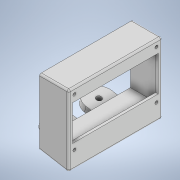
# Autodesk Inventor part: caica display
Saved by Autodesk Inventor 2022 (Build 260153000, 153)
## iProperties
Created: 2022-03-11
Part Number: caica display
Material: Genérico
Document SubType Name: Modeling
Designer: Guilherme
Density: 1 g/cm^3
Appearance: Padrão
Author: Guilherme
Autodesk Inventor part; units mm, degrees
ref_plane "YZ Plane" through (0, 0, 0) normal (1, 0, 0) x (0, 1, 0)
ref_plane "XZ Plane" through (0, 0, 0) normal (0, 1, 0) x (-1, 0, 0)
ref_plane "XY Plane" through (0, 0, 0) normal (0, 0, 1) x (1, 0, 0)
sketch "Esboço1" plane through (0, 0, 0) normal (1, 0, 0) x (0, 1, 0)
  line L0 (-31, 50) -> (31, 50)
  line L1 (31, 50) -> (31, -50)
  line L2 (31, -50) -> (-31, -50)
  line L3 (-31, -50) -> (-31, 50)
  line L4 (-31, 50) -> (31, -50) construction
  line L5 (31, 50) -> (-31, -50) construction
  point P0 (0, 0)
  dimension "d0" = 62
  dimension "d1" = 100
  constraints: 12 end point, 2 midpoint, 2 parallel, 1 horizontal, 1 perpendicular
  measures "d0" distance of L1.end L2.end
  measures "d1" distance of L0.end L1.end
extrude "Extrusão1" add sketch "Esboço1" along normal blind 3
sketch "Esboço4" plane through (0, 0, 0) normal (-1, 0, 0) x (0, 0, 1)
  line L0 (-50, 31) -> (50, 31) projected
  line L1 (-50, -31) -> (50, -31)
  line L2 (50, -31) -> (50, 31)
  line L3 (50, 31) -> (-50, 31)
  line L4 (-50, 31) -> (-50, -31)
  line L5 (-50, -31) -> (50, 31) construction
  line L6 (50, -31) -> (-50, 31) construction
  line L7 (-53, -34) -> (53, -34)
  line L8 (53, -34) -> (53, 34)
  line L9 (53, 34) -> (-53, 34)
  line L10 (-53, 34) -> (-53, -34)
  line L11 (-53, -34) -> (53, 34) construction
  line L12 (53, -34) -> (-53, 34) construction
  point P0 (0, 0)
  dimension "d16" = 106
  dimension "d17" = 68
  constraints: 24 end point, 4 midpoint, 4 parallel, 2 horizontal, 2 perpendicular
  measures "d16" distance of L9.end L8.end
  measures "d17" distance of L8.end L7.end
extrude "Extrusão3" add sketch "Esboço4" along normal blind 30 and the other way blind 3
sketch "Esboço5" plane through (0, 0, 0) normal (-1, 0, 0) x (0, 0, 1)
  line L0 (-49.0345, -29.972) -> (49.0345, -29.972)
  line L1 (49.0345, -29.972) -> (49.0345, 29.972)
  line L2 (49.0345, 29.972) -> (-49.0345, 29.972)
  line L3 (-49.0345, 29.972) -> (-49.0345, -29.972)
  line L4 (-49.0345, -29.972) -> (49.0345, 29.972) construction
  line L5 (49.0345, -29.972) -> (-49.0345, 29.972) construction
  line L6 (-48.55, -20) -> (48.55, -20)
  line L7 (48.55, -20) -> (48.55, 20)
  line L8 (48.55, 20) -> (-48.55, 20)
  line L9 (-48.55, 20) -> (-48.55, -20)
  line L10 (-48.55, -20) -> (48.55, 20) construction
  line L11 (48.55, -20) -> (-48.55, 20) construction
  circle A0 centre (46.4815, 27.305) radius 1.6765
  circle A1 centre (-46.4825, 27.305) radius 1.6765
  circle A2 centre (46.4815, -27.305) radius 1.6765
  circle A3 centre (-46.4825, -27.305) radius 1.6765
  point P0 (0, 0)
  dimension "d22" = 98.069
  dimension "d23" = 59.944
  dimension "d24" = 97.1
  dimension "d25" = 40
  dimension "d26" = 3.353
  dimension "d27" = 2.667
  dimension "d28" = 2.553
  dimension "d31" = 92.964
  dimension "d34" = 54.61
  constraints: 24 end point, 4 centre point, 4 midpoint, 4 parallel, 3 horizontal, 2 perpendicular, 1 vertical, 6 other
  measures "d22" distance of L2.end L1.end
  measures "d23" distance of L1.end L0.end
  measures "d24" distance of L8.end L7.end
  measures "d25" distance of L7.end L6.end
  measures "d26" diameter of A0
  measures "d27" distance from line of L2 A0.centre
  measures "d28" distance from line of L1 A0.centre
  measures "d31" distance of A0.centre A1.centre
  measures "d34" distance of A0.centre A2.centre
extrude "Extrusão4" cut sketch "Esboço5" against normal blind 30 contours L9 L8 L7 L6 | A0 | A1 | A2 | A3
sketch "Esboço20" plane through (-30, 34, 53) normal (0, 0, 1) x (1, 0, 0)
  line L0 (0, -68) -> (0, 0) projected
  line L1 (0, -68) -> (33, -68)
  line L2 (33, -68) -> (33, -75)
  line L3 (0, -75) -> (0, -68)
  line L4 (0, -75) -> (33, -80.8188)
  line L5 (0, -75) -> (34.0016, -75) construction
  line L6 (33, -75) -> (33, -80.8188)
  point P0 (30, -34)
  dimension "d110" = 10
  constraints: 12 end point, 2 horizontal, 2 perpendicular, 1 parallel
  measures "d110" angle of L4 L5
extrude "Extrusão16" add sketch "Esboço20" against normal blind 106
sketch "Esboço23" plane through (-30, 34, 53) normal (0, 0, 1) x (1, 0, 0)
  line L0 (0, 0) -> (0, -75) projected
  line L1 (0, -75) -> (-24.6202, -70.6588)
  line L2 (0, -75) -> (25, -75) construction
  line L3 (-24.6202, -70.6588) -> (-23.4047, -63.7651)
  line L4 (-23.4047, -63.7651) -> (0, -67.892)
  line L5 (0, -67.892) -> (0, -75)
  point P0 (30, -34)
  dimension "d122" = 25
  dimension "d123" = 170
  dimension "d124" = 7
  constraints: 10 end point, 2 perpendicular, 1 equal length, 1 horizontal, 1 point on line, 1 vertical
  measures "d122" distance of L0.end L1.end
  measures "d123" angle of L2 L1
  measures "d124" distance of L1.end L3.end
extrude "Extrusão18" add sketch "Esboço23" against normal blind 106
sketch "Esboço24" plane through (-30, 34, -53) normal (0, 1, 0) x (1, 0, 0)
  line L0 (0, -103) -> (0, -3) projected
  line L1 (0, -15) -> (-28.0822, -15)
  line L2 (-28.0822, -45) -> (0, -45)
  line L3 (0, -45) -> (0, -15)
  line L4 (0, -61) -> (-33.5512, -61)
  line L5 (-33.5512, -91) -> (0, -91)
  line L6 (0, -91) -> (0, -61)
  line L7 (-23.4047, 0) -> (0, 0) projected
  line L8 (0, -106) -> (-23.4047, -106) projected
  line L9 (0, 0) -> (-32.176, 0)
  line L10 (-32.176, 0) -> (-32.176, -15)
  line L11 (-32.176, -15) -> (0, -15)
  line L12 (0, -15) -> (0, 0)
  line L13 (0, -45) -> (-41.5151, -45)
  line L14 (-41.5151, -45) -> (-41.5151, -61)
  line L15 (-41.5151, -61) -> (0, -61)
  line L16 (0, -61) -> (0, -45)
  line L17 (0, -91) -> (-36.7607, -91)
  line L18 (-36.7607, -91) -> (-36.7607, -106)
  line L19 (-36.7607, -106) -> (0, -106)
  line L20 (0, -106) -> (0, -91)
  point P0 (30, -53)
  point P1 (0, -91)
  point P2 (0, -61)
  point P3 (0, -45)
  point P4 (-28.0822, -45)
  point P5 (-28.0822, -15)
  constraints: 36 end point, 8 parallel, 5 horizontal, 3 perpendicular, 2 point on line
extrude "Extrusão19" cut sketch "Esboço24" against normal blind 106
fillet "Arredondamento7" radius 15 4 edges at (-54.0124, -33.212, -38) (-54.0124, -33.212, -8) (-54.0124, -33.212, 8) (-54.0124, -33.212, 38)
sketch "Esboço25" plane through (-30, -33.892, -8) normal (0.1736482, 0.9848078, 0) x (0.9848078, -0.1736482, 0)
  arc A0 (-8.7657, 30) -> (-8.7657, 0) centre (-8.7657, 15) ccw projected
  circle A1 centre (-8.7657, 15) radius 3.05
  arc A2 (-8.7657, -16) -> (-8.7657, -46) centre (-8.7657, -31) ccw projected
  circle A3 centre (-8.7657, -31) radius 3.05
  point P0 (23.6589, -8)
  dimension "d134" = 6.1
  dimension "d135" = 6.1
  constraints: 2 centre point, 2 coincident
  measures "d134" diameter of A1
  measures "d135" diameter of A3
extrude "Extrusão20" cut sketch "Esboço25" against normal blind 106
fillet "Arredondamento8" radius 2 4 edges at (-13.5, 34, 53) (-13.5, -43.9094, 53) (-13.5, 34, -53) (-13.5, -43.9094, -53)
fillet "Arredondamento9" radius 2 8 edges at (3, 33.4142, 52.4142) (3, -6.394, 53) (3, -46.224, 52.4142) (3, -46.8188, 0) (3, -46.224, -52.4142) (3, -6.394, -53) (3, 33.4142, -52.4142) (3, 34, 0)
